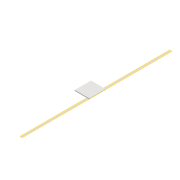
# Autodesk Inventor part: PlacaInferior
Saved by Autodesk Inventor 2021 (Build 250183000, 183)
## iProperties
Created: 2021-05-05
Part Number: PlacaInferior
Material: Generic
Document SubType Name: Modeling
Designer: Santiago Suárez
Mass: 789.888 g
Surface Area: 1439.84 cm^2
Volume: 789.888 cm^3
Density: 1 g/cm^3
Appearance: Default
Author: Santiago Suárez
Autodesk Inventor part; units mm, degrees
ref_plane "YZ Plane" through (0, 0, 0) normal (1, 0, 0) x (0, 1, 0)
ref_plane "XZ Plane" through (0, 0, 0) normal (0, 1, 0) x (-1, 0, 0)
ref_plane "XY Plane" through (0, 0, 0) normal (0, 0, 1) x (1, 0, 0)
ref_plane "Work Plane1" through (1104.5696, 91.5553, 211.8164) normal (0, 1, 0) x (-1, 0, 0)
sketch "Sketch1" plane through (1104.5696, 91.5553, 211.8164) normal (0, 1, 0) x (-1, 0, 0)
  arc A0 (57.6551, 1254.9955) -> (57.6551, 1150.0245) centre (104.395, 1202.51) ccw projected
  line L0 (-26.3951, 1291) -> (123.6049, 1291) projected
  line L1 (123.6049, 1019) -> (-26.3951, 1019) projected
  line L2 (-26.3951, 1249) -> (-26.3951, 1291) projected
  line L3 (169.6049, 2289.9999) -> (169.6049, 25.0001) projected
  line L4 (169.6049, 1019) -> (169.6049, 1291.0001)
  line L5 (-72.3951, 25.0001) -> (-72.3951, 2289.9999) projected
  line L6 (169.6049, 1291.0001) -> (-72.3951, 1291.0001)
  line L7 (169.6049, 1019) -> (-72.3951, 1019)
  line L8 (-72.3951, 1291.0001) -> (-72.3951, 1019)
  point P0 (1104.5696, -211.8164)
  point P1 (154, 1291)
  point P2 (4, 1291)
  constraints: 8 end point, 5 point on line, 2 collinear, 2 perpendicular
extrude "Extrusion1" add sketch "Sketch1" along normal blind 12
body "Solid1"
